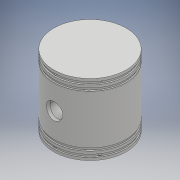
# Autodesk Inventor part: Хрень от поршня
Saved by Autodesk Inventor 2018 (Build 220112000, 112)
## iProperties
Created: 2020-04-16
Part Number: Хрень от поршня
Material: Типовые
Document SubType Name: Modeling
Designer: 2000
Density: 1 g/cm^3
Appearance: По умолчанию
Mass: 21.7426 g
Surface Area: 237.319 cm^2
Volume: 21.7426 cm^3
Author: 2000
Autodesk Inventor part; units mm, degrees
ref_plane "YZ Plane" through (0, 0, 0) normal (1, 0, 0) x (0, 1, 0)
ref_plane "XZ Plane" through (0, 0, 0) normal (0, 1, 0) x (-1, 0, 0)
ref_plane "XY Plane" through (0, 0, 0) normal (0, 0, 1) x (1, 0, 0)
sketch "Эскиз1" plane through (0, 0, 0) normal (0, 0, 1) x (1, 0, 0)
  circle A0 centre (0, 0) radius 26.5
  dimension "d0" = 53
  constraints: 1 centre point, 1 coincident
  measures "d0" diameter of A0
extrude "Выдавливание1" add sketch "Эскиз1" along normal blind 2
sketch "Эскиз2" plane through (0, 0, 2) normal (0, 0, 1) x (1, 0, 0)
  circle A0 centre (0, 0) radius 26.5 projected
  circle A1 centre (0, 0) radius 25.5
  dimension "d3" = 51
  constraints: 1 centre point, 1 coincident
  measures "d3" diameter of A1
extrude "Выдавливание2" add sketch "Эскиз2" along normal blind 2 contours A1
sketch "Эскиз3" plane through (0, 0, 4) normal (0, 0, 1) x (1, 0, 0)
  circle A0 centre (0, 0) radius 26.5
  dimension "d6" = 53
  constraints: 1 centre point, 1 coincident
  measures "d6" diameter of A0
extrude "Выдавливание3" add sketch "Эскиз3" along normal blind 2
sketch "Эскиз4" plane through (0, 0, 6) normal (0, 0, 1) x (1, 0, 0)
  circle A0 centre (0, 0) radius 25.5
  dimension "d9" = 51
  constraints: 1 centre point, 1 coincident
  measures "d9" diameter of A0
extrude "Выдавливание4" add sketch "Эскиз4" along normal blind 2
sketch "Эскиз5" plane through (0, 0, 8) normal (0, 0, 1) x (1, 0, 0)
  circle A0 centre (0, 0) radius 26.5
  dimension "d12" = 53
  constraints: 1 centre point, 1 coincident
  measures "d12" diameter of A0
extrude "Выдавливание5" add sketch "Эскиз5" along normal blind 36
sketch "Эскиз6" plane through (0, 0, 44) normal (0, 0, 1) x (1, 0, 0)
  circle A0 centre (0, 0) radius 25.5
  dimension "d15" = 51
  constraints: 1 centre point, 1 coincident
  measures "d15" diameter of A0
extrude "Выдавливание6" add sketch "Эскиз6" along normal blind 2
sketch "Эскиз7" plane through (0, 0, 46) normal (0, 0, 1) x (1, 0, 0)
  circle A0 centre (0, 0) radius 26.5
  dimension "d18" = 53
  constraints: 1 centre point, 1 coincident
  measures "d18" diameter of A0
extrude "Выдавливание7" add sketch "Эскиз7" along normal blind 2
sketch "Эскиз8" plane through (0, 0, 48) normal (0, 0, 1) x (1, 0, 0)
  circle A0 centre (0, 0) radius 25.5
  dimension "d21" = 51
  constraints: 1 centre point, 1 coincident
  measures "d21" diameter of A0
extrude "Выдавливание8" add sketch "Эскиз8" along normal blind 2
sketch "Эскиз9" plane through (0, 0, 50) normal (0, 0, 1) x (1, 0, 0)
  circle A0 centre (0, 0) radius 26.5
  dimension "d24" = 53
  constraints: 1 centre point, 1 coincident
  measures "d24" diameter of A0
extrude "Выдавливание9" add sketch "Эскиз9" along normal blind 2
sketch "Эскиз10" plane through (0, 0, 0) normal (0, 0, -1) x (-1, 0, 0)
  circle A0 centre (0, 0) radius 24
  dimension "d27" = 48
  constraints: 1 centre point, 1 coincident
  measures "d27" diameter of A0
extrude "Выдавливание10" cut sketch "Эскиз10" against normal blind 51
sketch "Эскиз11" plane through (0, 0, 0) normal (0, 1, 0) x (-1, 0, 0)
  circle A0 centre (0, 26) radius 6
  point P0 (0, 0)
  dimension "d30" = 12
  dimension "d31" = 26
  constraints: 1 centre point, 1 vertical alignment
  measures "d30" diameter of A0
  measures "d31" distance of A0.centre point (0, 0)
extrude "Выдавливание11" cut sketch "Эскиз11" along normal mid plane 53
sketch "Эскиз12" plane through (0, 0, 0) normal (0, 1, 0) x (-1, 0, 0)
  circle A0 centre (0, 26) radius 7.5
  spline S0 degree 5 poles (6, 26) (6, 26.7046) (5.8967, 27.4078) (5.6901, 28.1014) (5.3757, 28.7714) (4.5022, 30.0423) (3.9311, 30.6487) (3.2223, 31.1833) (2.3717, 31.6011) (0.5045, 32.0494) (-0.4623, 32.0994) (-1.423, 31.9428) (-2.2855, 31.6087) (-3.6919, 30.7967) (-4.2734, 30.3077) (-4.75, 29.7634) (-5.1282, 29.1855) (-5.8201, 27.7348) (-6.0438, 26.8384) (-6.0999, 25.9282) (-5.9907, 25.0212) (-5.4563, 23.3762) (-5.0711, 22.6327) (-4.5445, 21.9309) (-3.8566, 21.2984) (-2.2855, 20.3913) (-1.423, 20.0572) (-0.4623, 19.9006) (0.5045, 19.9506) (2.255, 20.3709) (3.0177, 20.7192) (3.674, 21.1666) (4.2201, 21.6773) (5.2119, 22.902) (5.6095, 23.6444) (5.8699, 24.4202) (6, 25.2089) (6, 26) knots 0 0 0 0 0 0 0.107622 0.107622 0.107622 0.107622 0.21813 0.21813 0.21813 0.21813 0.320117 0.320117 0.320117 0.320117 0.41887 0.41887 0.41887 0.41887 0.557915 0.557915 0.557915 0.557915 0.680187 0.680187 0.680187 0.680187 0.782186 0.782186 0.782186 0.782186 0.879429 0.879429 0.879429 0.879429 1 1 1 1 1 1 projected
  point P0 (0, 0)
  dimension "d34" = 15
  dimension "d35" = 26
  constraints: 1 centre point, 1 vertical alignment, 1 other
  measures "d34" diameter of A0
  measures "d35" distance of point (0, 0) A0.centre
extrude "Выдавливание12" add sketch "Эскиз12" along normal mid plane 49
sketch "Эскиз13" plane through (0, 0, 0) normal (0, 0, -1) x (-1, 0, 0)
  line L0 (-11, 14.5) -> (13, 14.5)
  line L1 (13, 14.5) -> (13, -14.5)
  line L2 (13, -14.5) -> (-11, -14.5)
  line L3 (-11, -14.5) -> (-11, 14.5)
  circle A0 centre (0, 0) radius 26.5 projected
  dimension "d40" = 24
  dimension "d41" = 13
  dimension "d42" = 12
  dimension "d44" = 12
  constraints: 8 end point, 2 parallel, 1 horizontal, 1 perpendicular
  measures "d40" distance between parallel lines of L1 L3
  measures "d41" distance from line of point (0, 0) L1
  measures "d42" distance edge to line of A0 L0
  measures "d44" distance edge to line of A0 L2
extrude "Выдавливание13" cut sketch "Эскиз13" against normal blind 49 contours L0 L1 L2 L3
sketch "Эскиз14" plane through (0, 0, 0) normal (1, 0, 0) x (0, 1, 0)
  circle A0 centre (14, 3) radius 0.75
  circle A1 centre (-14, 3) radius 0.75
  point P0 (0, 0)
  dimension "d47" = 1.5
  dimension "d48" = 1.5
  dimension "d49" = 3
  dimension "d50" = 3
  dimension "d51" = 14
  dimension "d52" = 14
  constraints: 2 centre point
  measures "d47" diameter of A0
  measures "d48" diameter of A1
  measures "d49" vertical distance of A0.centre point (0, 0)
  measures "d50" vertical distance of point (0, 0) A1.centre
  measures "d51" horizontal distance of point (0, 0) A0.centre
  measures "d52" horizontal distance of A1.centre point (0, 0)
extrude "Выдавливание14" cut sketch "Эскиз14" along normal mid plane 44
sketch "Эскиз15" plane through (0, 0, 0) normal (0, 1, 0) x (-1, 0, 0)
  circle A0 centre (0, 3) radius 0.75
  point P0 (0, 0)
  dimension "d55" = 1.5
  dimension "d56" = 3
  constraints: 1 centre point, 1 vertical alignment
  measures "d55" diameter of A0
  measures "d56" distance of point (0, 0) A0.centre
extrude "Выдавливание15" cut sketch "Эскиз15" along normal mid plane 53.75
sketch "Эскиз16" plane through (0, 0, 0) normal (0, 1, 0) x (-1, 0, 0)
  circle A0 centre (0, 49) radius 0.75
  point P0 (0, 0)
  dimension "d59" = 1.5
  dimension "d60" = 49
  constraints: 1 centre point, 1 vertical alignment
  measures "d59" diameter of A0
  measures "d60" distance of point (0, 0) A0.centre
extrude "Выдавливание16" cut sketch "Эскиз16" along normal mid plane 53.75
sketch "Эскиз17" plane through (0, 0, 0) normal (1, 0, 0) x (0, 1, 0)
  circle A0 centre (-14, 49) radius 0.75
  circle A1 centre (14, 49) radius 0.75
  point P0 (0, 0)
  dimension "d63" = 1.5
  dimension "d64" = 1.5
  dimension "d65" = 49
  dimension "d66" = 49
  dimension "d67" = 14
  dimension "d68" = 14
  constraints: 2 centre point
  measures "d63" diameter of A0
  measures "d64" diameter of A1
  measures "d65" vertical distance of point (0, 0) A0.centre
  measures "d66" vertical distance of point (0, 0) A1.centre
  measures "d67" horizontal distance of point (0, 0) A1.centre
  measures "d68" horizontal distance of point (0, 0) A0.centre
extrude "Выдавливание17" cut sketch "Эскиз17" along normal mid plane 45.5
fillet "Сопряжение1" radius 2.5 1 edges at (7.5, 22.798, 26.011)
fillet "Сопряжение2" radius 2.5 1 edges at (7.5, -22.798, 26.011)
